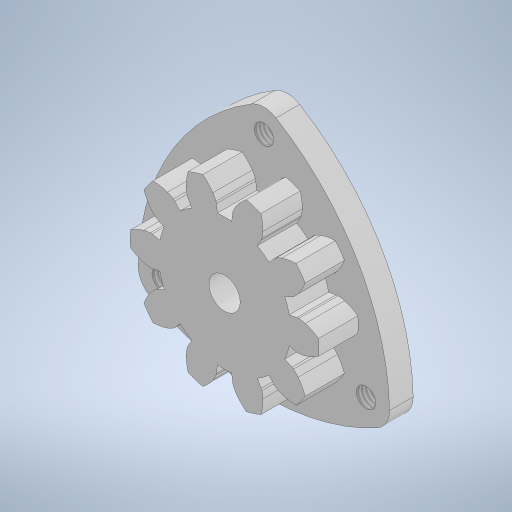
# Autodesk Inventor part: 多段ギアm2z10t8
Saved by Autodesk Inventor 2023 (Build 270158030, 158C)
## iProperties
Created: 2022-01-10
Part Number: 多段ギアm2z10t8
Material: Generic
Document SubType Name: Modeling
Designer: acps
Density: 1 g/cm^3
Appearance: Default
Author: acps
Autodesk Inventor part; units mm, degrees
ref_plane "YZ Plane" through (0, 0, 0) normal (1, 0, 0) x (0, 1, 0)
ref_plane "XZ Plane" through (0, 0, 0) normal (0, 1, 0) x (-1, 0, 0)
ref_plane "XY Plane" through (0, 0, 0) normal (0, 0, 1) x (1, 0, 0)
sketch "Sketch1" plane through (0, 0, 0) normal (0, 0, 1) x (1, 0, 0)
  arc A0 (1.0889, 9.5754) -> (1.0261, 9.3407) centre (2.2089, 9.1504) ccw
  arc A1 (1.4739, 10.3184) -> (1.0889, 9.5754) centre (4.2282, 8.4196) ccw
  arc A2 (2.7641, 11.6773) -> (1.4739, 10.3184) centre (6.4046, 6.9293) ccw
  arc A3 (-4.7474, 8.3867) -> (-4.6602, 8.16) centre (-3.5914, 8.7012) ccw
  arc A4 (-4.8726, 9.2141) -> (-4.7474, 8.3867) centre (-1.5283, 9.2968) ccw
  arc A5 (-4.6276, 11.0718) -> (-4.8726, 9.2141) centre (1.1085, 9.3704) ccw
  arc A6 (-8.7703, 3.9945) -> (-8.5665, 3.8624) centre (-8.0199, 4.9284) ccw
  arc A7 (-9.3579, 4.5903) -> (-8.7703, 3.9945) centre (-6.7009, 6.623) ccw
  arc A8 (-10.2517, 6.2373) -> (-9.3579, 4.5903) centre (-4.611, 8.2324) ccw
  arc A9 (-9.4432, -1.9234) -> (-9.2007, -1.9105) centre (-9.3851, -0.7268) ccw
  arc A10 (-10.2587, -1.7898) -> (-9.4432, -1.9234) centre (-9.3141, 1.4194) ccw
  arc A11 (-11.9599, -0.9797) -> (-10.2587, -1.7898) centre (-8.5693, 3.9498) ccw
  arc A12 (-6.5092, -7.1067) -> (-6.3205, -6.9537) centre (-7.1655, -6.1044) ccw
  arc A13 (-7.2574, -7.4814) -> (-6.5092, -7.1067) centre (-8.3696, -4.3263) ccw
  arc A14 (-9.0999, -7.8225) -> (-7.2574, -7.4814) centre (-9.2543, -1.8414) ccw
  arc A15 (-1.0889, -9.5754) -> (-1.0261, -9.3407) centre (-2.2089, -9.1504) ccw
  arc A16 (-1.4739, -10.3184) -> (-1.0889, -9.5754) centre (-4.2282, -8.4196) ccw
  arc A17 (-2.7641, -11.6773) -> (-1.4739, -10.3184) centre (-6.4046, -6.9293) ccw
  arc A18 (4.7474, -8.3867) -> (4.6602, -8.16) centre (3.5914, -8.7012) ccw
  arc A19 (4.8726, -9.2141) -> (4.7474, -8.3867) centre (1.5283, -9.2968) ccw
  arc A20 (4.6276, -11.0718) -> (4.8726, -9.2141) centre (-1.1085, -9.3704) ccw
  arc A21 (8.7703, -3.9945) -> (8.5665, -3.8624) centre (8.0199, -4.9284) ccw
  arc A22 (9.3579, -4.5903) -> (8.7703, -3.9945) centre (6.7009, -6.623) ccw
  arc A23 (10.2517, -6.2373) -> (9.3579, -4.5903) centre (4.611, -8.2324) ccw
  arc A24 (9.4432, 1.9234) -> (9.2007, 1.9105) centre (9.3851, 0.7268) ccw
  arc A25 (10.2688, 1.7868) -> (9.4432, 1.9234) centre (9.3141, -1.4194) ccw
  arc A26 (11.9599, 0.9797) -> (10.2688, 1.7868) centre (8.5693, -3.9498) ccw
  arc A27 (6.5092, 7.1067) -> (6.3205, 6.9537) centre (7.1655, 6.1044) ccw
  arc A28 (7.2574, 7.4814) -> (6.5092, 7.1067) centre (8.3696, 4.3263) ccw
  arc A29 (9.0999, 7.8225) -> (7.2574, 7.4814) centre (9.2543, 1.8414) ccw
  arc A30 (-1.0261, 9.3407) -> (-1.0889, 9.5754) centre (-2.2089, 9.1504) ccw
  arc A31 (-1.0889, 9.5754) -> (-1.4739, 10.3184) centre (-4.2282, 8.4196) ccw
  arc A32 (-1.4739, 10.3184) -> (-2.7641, 11.6773) centre (-6.4046, 6.9293) ccw
  arc A33 (-6.3205, 6.9537) -> (-6.5092, 7.1067) centre (-7.1655, 6.1044) ccw
  arc A34 (-6.5092, 7.1067) -> (-7.2574, 7.4814) centre (-8.3696, 4.3263) ccw
  arc A35 (-7.2574, 7.4814) -> (-9.0999, 7.8225) centre (-9.2543, 1.8414) ccw
  arc A36 (-9.2007, 1.9105) -> (-9.4432, 1.9234) centre (-9.3851, 0.7268) ccw
  arc A37 (-9.4432, 1.9234) -> (-10.2688, 1.7868) centre (-9.3141, -1.4194) ccw
  arc A38 (-10.2688, 1.7868) -> (-11.9599, 0.9797) centre (-8.5693, -3.9498) ccw
  arc A39 (-8.5665, -3.8624) -> (-8.7703, -3.9945) centre (-8.0199, -4.9284) ccw
  arc A40 (-8.7703, -3.9945) -> (-9.3579, -4.5903) centre (-6.7009, -6.623) ccw
  arc A41 (-9.3579, -4.5903) -> (-10.2517, -6.2373) centre (-4.611, -8.2324) ccw
  arc A42 (-4.6602, -8.16) -> (-4.7474, -8.3867) centre (-3.5914, -8.7012) ccw
  arc A43 (-4.7474, -8.3867) -> (-4.8726, -9.2141) centre (-1.5283, -9.2968) ccw
  arc A44 (-4.8726, -9.2141) -> (-4.6276, -11.0718) centre (1.1085, -9.3704) ccw
  arc A45 (1.0261, -9.3407) -> (1.0889, -9.5754) centre (2.2089, -9.1504) ccw
  arc A46 (1.0889, -9.5754) -> (1.4739, -10.3184) centre (4.2282, -8.4196) ccw
  arc A47 (1.4739, -10.3184) -> (2.7641, -11.6773) centre (6.4046, -6.9293) ccw
  arc A48 (6.3205, -6.9537) -> (6.5092, -7.1067) centre (7.1655, -6.1044) ccw
  arc A49 (6.5092, -7.1067) -> (7.2574, -7.4814) centre (8.3696, -4.3263) ccw
  arc A50 (7.2574, -7.4814) -> (9.0999, -7.8225) centre (9.2543, -1.8414) ccw
  arc A51 (9.2007, -1.9105) -> (9.4432, -1.9234) centre (9.3851, -0.7268) ccw
  arc A52 (9.4432, -1.9234) -> (10.2688, -1.7868) centre (9.3141, 1.4194) ccw
  arc A53 (10.2688, -1.7868) -> (11.9599, -0.9797) centre (8.5693, 3.9498) ccw
  arc A54 (8.5665, 3.8624) -> (8.7703, 3.9945) centre (8.0199, 4.9284) ccw
  arc A55 (8.7703, 3.9945) -> (9.3579, 4.5903) centre (6.7009, 6.623) ccw
  arc A56 (9.3579, 4.5903) -> (10.2517, 6.2373) centre (4.611, 8.2324) ccw
  arc A57 (4.6602, 8.16) -> (4.7474, 8.3867) centre (3.5914, 8.7012) ccw
  arc A58 (4.7474, 8.3867) -> (4.8726, 9.2141) centre (1.5283, 9.2968) ccw
  arc A59 (4.8726, 9.2141) -> (4.6276, 11.0718) centre (-1.1085, 9.3704) ccw
  arc A60 (0.9173, 8.3498) -> (-0.9173, 8.3498) centre (0, 0) ccw
  arc A61 (-4.1658, 7.2943) -> (-5.65, 6.2159) centre (0, 0) ccw
  arc A62 (-7.6576, 3.4526) -> (-8.2246, 1.7078) centre (0, 0) ccw
  arc A63 (-8.2246, -1.7078) -> (-7.6576, -3.4526) centre (0, 0) ccw
  arc A64 (-5.65, -6.2159) -> (-4.1658, -7.2943) centre (0, 0) ccw
  arc A65 (-0.9173, -8.3498) -> (0.9173, -8.3498) centre (0, 0) ccw
  arc A66 (4.1658, -7.2943) -> (5.65, -6.2159) centre (0, 0) ccw
  arc A67 (7.6576, -3.4526) -> (8.2246, -1.7078) centre (0, 0) ccw
  arc A68 (8.2246, 1.7078) -> (7.6576, 3.4526) centre (0, 0) ccw
  arc A69 (5.65, 6.2159) -> (4.1658, 7.2943) centre (0, 0) ccw
  arc A70 (-2.7641, 11.6773) -> (-4.6276, 11.0718) centre (0, 0) ccw
  arc A71 (-9.0999, 7.8225) -> (-10.2517, 6.2373) centre (0, 0) ccw
  arc A72 (-11.9599, 0.9797) -> (-11.9599, -0.9797) centre (0, 0) ccw
  arc A73 (-10.2517, -6.2373) -> (-9.0999, -7.8225) centre (0, 0) ccw
  arc A74 (-4.6276, -11.0718) -> (-2.7641, -11.6773) centre (0, 0) ccw
  arc A75 (2.7641, -11.6773) -> (4.6276, -11.0718) centre (0, 0) ccw
  arc A76 (9.0999, -7.8225) -> (10.2517, -6.2373) centre (0, 0) ccw
  arc A77 (11.9599, -0.9797) -> (11.9599, 0.9797) centre (0, 0) ccw
  arc A78 (10.2517, 6.2373) -> (9.0999, 7.8225) centre (0, 0) ccw
  arc A79 (4.6276, 11.0718) -> (2.7641, 11.6773) centre (0, 0) ccw
  line L0 (0.9173, 8.3498) -> (1.0261, 9.3407)
  line L1 (-4.1658, 7.2943) -> (-4.6602, 8.16)
  line L2 (-7.6576, 3.4526) -> (-8.5665, 3.8624)
  line L3 (-8.2246, -1.7078) -> (-9.2007, -1.9105)
  line L4 (-5.65, -6.2159) -> (-6.3205, -6.9537)
  line L5 (-0.9173, -8.3498) -> (-1.0261, -9.3407)
  line L6 (4.1658, -7.2943) -> (4.6602, -8.16)
  line L7 (7.6576, -3.4526) -> (8.5665, -3.8624)
  line L8 (8.2246, 1.7078) -> (9.2007, 1.9105)
  line L9 (5.65, 6.2159) -> (6.3205, 6.9537)
  line L10 (-0.9173, 8.3498) -> (-1.0261, 9.3407)
  line L11 (-5.65, 6.2159) -> (-6.3205, 6.9537)
  line L12 (-8.2246, 1.7078) -> (-9.2007, 1.9105)
  line L13 (-7.6576, -3.4526) -> (-8.5665, -3.8624)
  line L14 (-4.1658, -7.2943) -> (-4.6602, -8.16)
  line L15 (0.9173, -8.3498) -> (1.0261, -9.3407)
  line L16 (5.65, -6.2159) -> (6.3205, -6.9537)
  line L17 (8.2246, -1.7078) -> (9.2007, -1.9105)
  line L18 (7.6576, 3.4526) -> (8.5665, 3.8624)
  line L19 (4.1658, 7.2943) -> (4.6602, 8.16)
  circle A80 centre (0, 0) radius 2
  dimension "d34" = 4
  constraints: 160 point on circle, 81 centre point, 40 end point, 1 coincident
  measures "d34" diameter of A80
extrude "Extrusion1" add sketch "Sketch1" along normal blind 5
sketch "Sketch3" plane through (0, 0, 0) normal (0, 0, -1) x (-1, 0, 0)
  circle A0 centre (-12.9904, -7.5) radius 1.25
  circle A1 centre (12.9904, -7.5) radius 1.25
  circle A2 centre (0, 15) radius 1.25
  circle A3 centre (0, 0) radius 20.05 construction
  circle A4 centre (0, 0) radius 18.25 construction
  circle A5 centre (-12.9904, -7.5) radius 3.25 construction
  circle A6 centre (-12.9904, -7.5) radius 3
  circle A7 centre (12.9904, -7.5) radius 3
  circle A8 centre (0, 15) radius 3
  arc A9 (-1.5559, 17.565) -> (-15.9897, -7.435) centre (14.0033, -8.0848) ccw
  arc A10 (-14.4338, -10.13) -> (14.4338, -10.13) centre (0, 16.1696) ccw
  arc A11 (15.9897, -7.435) -> (1.5559, 17.565) centre (-14.0033, -8.0848) ccw
  circle A12 centre (0, 0) radius 2
  point P0 (15.9897, -7.435)
  point P1 (1.5559, 17.565)
  point P2 (-14.4338, -10.13)
  point P3 (14.4338, -10.13)
  dimension "d14" = 6
  dimension "d18" = 6
  dimension "d3" = 2.5
  dimension "d6" = 360
  dimension "d9" = 40.1
  dimension "d10" = 36.5
  dimension "d11" = 6.5
  dimension "d17" = 6
  dimension "d19" = 30
  dimension "d22" = 360
  dimension "d33" = 4
  constraints: 11 centre point, 7 coincident, 6 point on circle, 1 horizontal alignment, 1 tangent, 28 other
  measures "d3" diameter of A0
  measures "d9" diameter of A3
  measures "d10" diameter of A4
  measures "d11" diameter of A5
  measures "d17" diameter of A7
  measures "d19" radius of A9
  measures "d33" diameter of A12
extrude "Extrusion2" add sketch "Sketch3" along normal blind 3
thread "Thread1" size "M3x0.5" class "6H" standard "ANSI Metric M Profile" full length
thread "Thread2" size "M3x0.5" class "6H" standard "ANSI Metric M Profile" full length
thread "Thread3" size "M3x0.5" class "6H" standard "ANSI Metric M Profile" full length
body "Solid1"
